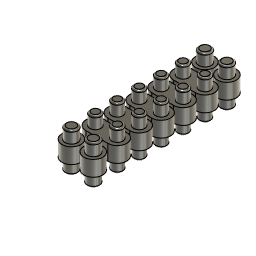
seperators v5 (Autodesk Fusion 360 design; units mm, degrees)
Autodesk Fusion 360 part; units mm, degrees
note: some values were not read from the file. Set by a fixed rule: which face or edge a step refers to.
sketch "Sketch1" plane through (0, 0, 0) normal (0, 0, 1) x (1, 0, 0)
  circle A0 centre (0, 0) radius 1.6
  dimension "d1" = 3.2
  constraint coincident A0.centre origin
  measures "d1" diameter of A0
extrude "Extrude1" add sketch "Sketch1" along normal blind 11.5 makes body 1
fillet "Fillet1" radius 0.5 2 edges at (-1.4917, -0.5786, 11.5) (-1.4917, -0.5786, 0) on bodies 1
ref_plane "WorkPlane1" through (0, 0, 5.75) normal (0, 0, 1) x (1, 0, 0)
sketch "Sketch2" plane through (0, 0, 5.75) normal (0, 0, 1) x (1, 0, 0)
  circle A0 centre (0, 0) radius 2.75
  dimension "d4" = 5.5
  constraint coincident A0.centre origin
  measures "d4" diameter of A0
extrude "Extrude2" add sketch "Sketch2" along normal blind 2.25 and the other way blind 2.25 bodies 1
copy_body "CopyPasteBodies1" bodies 1 makes body 2
move_body "Move1" bodies 2 to x (1, 0, 0) y (0, 1, 0) z (0, 0, 1) at (0, 20, 0)
copy_body "CopyPasteBodies2" bodies 2 makes body 3
move_body "Move2" bodies 3 to x (1, 0, 0) y (0, 1, 0) z (0, 0, 1) at (6.4, 0, 0)
sketch "Sketch3" plane through (0, 0, 8) normal (0, 0, 1) x (-1, 0, 0)
  circle A0 centre (-6.4, -20) radius 2.75
  circle A1 centre (-6.4, -20) radius 1.6
  line L0 (-6.4195, -17.2501) -> (-0.0195, -17.2501)
  line L1 (-0.0195, -17.2501) -> (-0.0195, -22.7083)
  line L2 (-0.0195, -22.7083) -> (-6.4195, -22.7083)
  line L3 (-6.4195, -22.7083) -> (-6.4195, -17.2501)
  dimension "d9" = 6.4
  constraint horizontal L0
  constraint vertical L1
  constraint horizontal L2
  constraint vertical L3
  constraint coincident A0 L0.start
  measures "d9" distance of L0.start L0.end
extrude "Extrude3" add sketch "Sketch3" against normal blind 4.5 contours A0 L0 L1 L2 bodies 2 3
move_body "Move3" bodies 1 to x (1, 0, 0) y (0, 1, 0) z (0, 0, 1) at (0, 13, 0)
copy_body "CopyPasteBodies3" bodies 1 makes body 4
move_body "Move4" bodies 4 to x (1, 0, 0) y (0, 1, 0) z (0, 0, 1) at (6.4, 0, 0)
copy_body "CopyPasteBodies4" bodies 2 makes body 5
move_body "Move5" bodies 5 to x (1, 0, 0) y (0, 1, 0) z (0, 0, 1) at (0, 6.4, 0)
copy_body "CopyPasteBodies5" bodies 5 2 makes body 6 makes body 7
move_body "Move6" bodies 6 7 to x (1, 0, 0) y (0, 1, 0) z (0, 0, 1) at (0, 12.8, 0)
copy_body "CopyPasteBodies6" bodies 6 makes body 8
move_body "Move7" bodies 8 to x (1, 0, 0) y (0, 1, 0) z (0, 0, 1) at (0, 6.4, 0)
copy_body "CopyPasteBodies7" bodies 4 1 makes body 9 makes body 10
move_body "Move8" bodies 9 10 to x (1, 0, 0) y (0, 1, 0) z (0, 0, 1) at (0, 39, 0)
move_face "OffsetFaces1" offset 0.2 1 faces at (7.992, 52.1593, 2.5) on bodies 9
move_face "OffsetFaces2" offset 0.2 1 faces at (7.992, 52.1593, 9) on bodies 9
move_face "OffsetFaces3" offset 0.2 1 faces at (1.592, 52.1593, 9) on bodies 10
move_face "OffsetFaces4" offset 0.2 1 faces at (1.592, 13.1593, 9) on bodies 1
move_face "OffsetFaces5" offset 0.2 1 faces at (7.992, 13.1593, 9) on bodies 4
move_face "OffsetFaces6" offset 0.2 1 faces at (7.992, 13.1593, 2.5) on bodies 4
move_face "OffsetFaces7" offset 0.2 1 faces at (1.592, 13.1593, 2.5) on bodies 1
